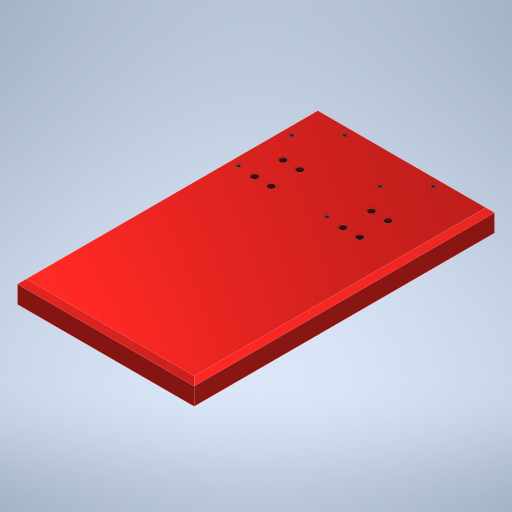
# Autodesk Inventor part: Carrier Wirebonding Plate
Saved by Autodesk Inventor 2023 (Build 270158000, 158)
## iProperties
Created: 2023-03-15
Part Number: Carrier Wirebonding Plate
Material: Aluminum, Anodized Red
Document SubType Name: Modeling
Designer: Caleb
Density: 2.7 g/cm^3
Appearance: Anodized - Red
Author: Caleb
Autodesk Inventor part; units mm, degrees
ref_plane "YZ Plane" through (0, 0, 0) normal (1, 0, 0) x (0, 1, 0)
ref_plane "XZ Plane" through (0, 0, 0) normal (0, 1, 0) x (-1, 0, 0)
ref_plane "XY Plane" through (0, 0, 0) normal (0, 0, 1) x (1, 0, 0)
sketch "Sketch1" plane through (0, 0, 0) normal (0, 1, 0) x (-1, 0, 0)
  line L0 (-63.5, -107.95) -> (63.5, -107.95)
  line L1 (63.5, -107.95) -> (63.5, 107.95)
  line L2 (63.5, 107.95) -> (-63.5, 107.95)
  line L3 (-63.5, 107.95) -> (-63.5, -107.95)
  line L4 (-63.5, -107.95) -> (63.5, 107.95) construction
  line L5 (63.5, -107.95) -> (-63.5, 107.95) construction
  point P0 (0, 0)
  dimension "d0" = 215.9
  dimension "d1" = 127
  constraints: 12 end point, 2 midpoint, 2 parallel, 1 horizontal, 1 perpendicular
  measures "d0" distance of L0.end L1.end
  measures "d1" distance of L1.end L2.end
extrude "Extrusion1" add sketch "Sketch1" along normal blind 15.75
sketch "Sketch2" plane through (0, 15.75, 0) normal (0, 1, 0) x (1, 0, 0)
  line L0 (-63.5, 107.95) -> (-63.5, -107.95) projected
  line L1 (63.5, 107.95) -> (-63.5, 107.95) projected
  point P0 (0, 0)
  point P1 (-54.61, 80.01)
  point P2 (-35.56, 99.06)
  point P3 (-54.61, 41.91)
  point P4 (8.89, 41.91)
  point P5 (27.94, 99.06)
  point P6 (8.89, 80.01)
  dimension "d4" = 8.89
  dimension "d5" = 8.89
  dimension "d7" = 19.05
  dimension "d8" = 19.05
  dimension "d16" = 38.1
  dimension "d29" = 63.5
  constraints: 1 horizontal, 1 vertical alignment, 3 other
  measures "d4" distance from line of L0 point (-54.61, 80.01)
  measures "d5" distance from line of L1 point (-35.56, 99.06)
  measures "d7" horizontal distance of point (-35.56, 99.06) point (-54.61, 80.01)
  measures "d8" horizontal distance of point (-54.61, 80.01) point (-35.56, 99.06)
  measures "d16" distance of point (-54.61, 80.01) point (-54.61, 41.91)
  measures "d29" distance of point (-54.61, 41.91) point (8.89, 41.91)
hole "Hole1" at (-54.61, 15.75, -80.01) at (-35.56, 15.75, -99.06) at (-54.61, 15.75, -41.91) at (27.94, 15.75, -99.06) at (8.89, 15.75, -80.01) at (8.89, 15.75, -41.91) direction (0, -1, 0) diameter 3.242 end through all thread size "M4x0.7" class "6H" standard "ANSI Metric M Profile"
sketch "Sketch3" plane through (0, 15.75, 0) normal (0, 1, 0) x (1, 0, 0)
  circle A0 centre (-42.1132, 41.0718) radius 2.5
  circle A1 centre (-42.1132, 61.5696) radius 2.5
  circle A2 centre (-30.1244, 61.5696) radius 2.5
  circle A3 centre (-30.1244, 41.0718) radius 2.5
  line L0 (-63.5, 107.95) -> (-63.5, -107.95) projected
  line L1 (63.5, 107.95) -> (-63.5, 107.95) projected
  circle A4 centre (21.3868, 41.0718) radius 2.5
  circle A5 centre (21.3868, 61.5696) radius 2.5
  circle A6 centre (33.3756, 61.5696) radius 2.5
  circle A7 centre (33.3756, 41.0718) radius 2.5
  point P0 (0, 0)
  dimension "d17" = 5
  dimension "d18" = 5
  dimension "d19" = 5
  dimension "d20" = 5
  dimension "d21" = 20.4978
  dimension "d22" = 11.9888
  dimension "d23" = 21.3868
  dimension "d24" = 46.3804
  dimension "d36" = 63.5
  constraints: 8 centre point, 2 horizontal alignment, 2 vertical alignment, 1 horizontal, 8 other
  measures "d17" diameter of A0
  measures "d18" diameter of A1
  measures "d19" diameter of A3
  measures "d20" diameter of A2
  measures "d21" distance of A3.centre A2.centre
  measures "d22" distance of A0.centre A3.centre
  measures "d23" distance from line of L0 A1.centre
  measures "d24" distance from line of L1 A1.centre
  measures "d36" distance of A0.centre A4.centre
extrude "Extrusion2" cut sketch "Sketch3" against normal through all
chamfer "Chamfer1" distance 3.175 angle 45 4 edges at (0, 15.75, 107.95) (63.5, 15.75, 0) (0, 15.75, -107.95) (-63.5, 15.75, 0)
equation "\"d18\" = d17"
equation "\"d19\" = d17"
equation "\"d20\" = d17"
body "Solid1"
